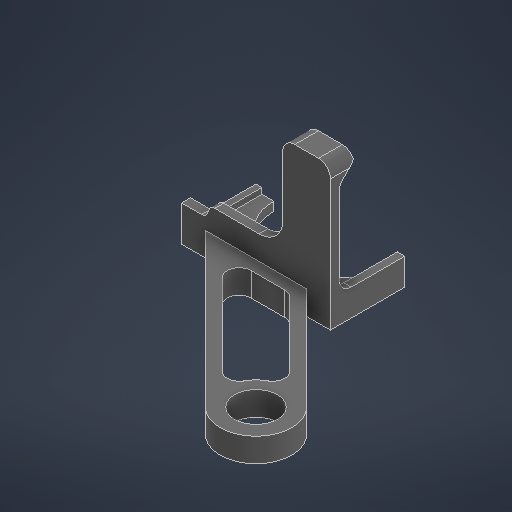
# Autodesk Inventor part: P_DroneCase
Saved by Autodesk Inventor 2026.2 (Build 302298000, 298)
## iProperties
Created: 2025-08-01
Part Number: P_DroneCase
Material: Generisch
Document SubType Name: Modeling
Designer: FAL
Density: 1 g/cm^3
Appearance: Vorgabe
Author: FAL
Autodesk Inventor part; units mm, degrees
ref_plane "YZ Plane" through (0, 0, 0) normal (1, 0, 0) x (0, 1, 0)
ref_plane "XZ Plane" through (0, 0, 0) normal (0, 1, 0) x (-1, 0, 0)
ref_plane "XY Plane" through (0, 0, 0) normal (0, 0, 1) x (1, 0, 0)
sketch "Skizze1" plane through (0, 0, 0) normal (0, 0, 1) x (1, 0, 0)
  line L0 (-25, 0) -> (25, 0)
  line L1 (25, 0) -> (25, -12.5)
  line L2 (25, -12.5) -> (-25, -12.5)
  line L3 (-25, -12.5) -> (-25, 0)
  line L4 (0, 0) -> (0, -12.5)
  dimension "d0" = 50
  dimension "d1" = 12.5
  constraints: 10 end point, 3 midpoint, 2 parallel, 1 horizontal, 1 perpendicular, 1 point on line
  measures "d0" distance of L1.end L2.end
  measures "d1" distance between parallel lines of L0 L2
extrude "Extrusion1" add sketch "Skizze1" along normal blind 24 contours L0 L1 L2 L4
sketch "Skizze24" plane through (0, 0, 0) normal (0, 0, 1) x (1, 0, 0)
  line L0 (0, 0) -> (33.9411, -33.9411) construction
  line L1 (4.2426, 4.2426) -> (38.1838, -29.6985)
  line L2 (29.6985, -38.1838) -> (-4.2426, -4.2426)
  arc A0 (4.2426, 4.2426) -> (-4.2426, -4.2426) centre (0, 0) ccw
  arc A1 (29.6985, -38.1838) -> (38.1838, -29.6985) centre (33.9411, -33.9411) ccw
  line L3 (0, 0) -> (0, -54.7704)
  line L4 (25, -12.5) -> (25, 0) projected
  line L5 (25, 0) -> (-45.4025, 0)
  point P0 (16.9706, -16.9706)
  point P1 (8.4853, 0)
  point P2 (-6, 0)
  point P3 (0, -8.4853)
  dimension "d137" = 45
  dimension "d138" = 48
  dimension "d139" = 12
  constraints: 12 end point, 4 point on circle, 4 tangent, 2 centre point, 1 horizontal, 1 midpoint, 1 parallel, 1 vertical
  measures "d137" angle of L3 L0
  measures "d138" distance of L0.start L0.end
  measures "d139" distance between parallel lines of L2 L1
extrude "Extrusion19" add sketch "Skizze24" along normal blind 4 contours L1 A1 L2 L3 L5
sketch "Skizze25" plane through (0, 0, 4) normal (0, 0, 1) x (1, 0, 0)
  arc A0 (29.6985, -38.1838) -> (38.1838, -29.6985) centre (33.9411, -33.9411) ccw projected
  circle A1 centre (33.9411, -33.9411) radius 3.575
  circle A2 centre (33.9411, -33.9411) radius 5.575
  line L0 (28.3667, -34.0236) -> (6.8431, -12.5)
  line L1 (0, -12.5) -> (25, -12.5) projected
  line L2 (18.1569, -12.5) -> (34.0236, -28.3667)
  line L3 (4.0147, -12.5) -> (29.6985, -38.1838) projected
  line L4 (38.1838, -29.6985) -> (20.9853, -12.5) projected
  line L5 (8.8431, -14.5) -> (20.1569, -14.5)
  point P0 (0, 0)
  point P1 (-35, -12.5)
  dimension "d142" = 7.15
  dimension "d143" = 2
  dimension "d144" = 2
  dimension "d145" = 2
  dimension "d149" = 2
  constraints: 6 end point, 4 parallel, 4 point on line, 2 centre point, 2 coincident, 2 point on circle
  measures "d142" diameter of A1
  measures "d143" distance between parallel lines of L3 L0
  measures "d144" distance between parallel lines of L4 L2
  measures "d145" radial gap between concentric circles of A1 A2
  measures "d149" distance between parallel lines of L1 L5
extrude "Extrusion20" cut sketch "Skizze25" against normal through all contours L5 L2 A2 L0 | A1
fillet "Rundung14" radius 2 4 edges at (28.3667, -34.0236, 2) (34.0236, -28.3667, 2) (8.8431, -14.5, 2) (20.1569, -14.5, 2)
sketch "Skizze26" plane through (25, -12.5, 0) normal (1, 0, 0) x (0, 0, -1)
  line L0 (0, 12.5) -> (-24, 12.5) projected
  line L1 (-24, 12.5) -> (-1.5, 12.5)
  line L2 (-1.5, 12.5) -> (-1.5, 1.5)
  line L3 (-1.5, 1.5) -> (-24, 1.5)
  line L4 (-24, 1.5) -> (-24, 12.5)
  line L5 (0, 0) -> (0, 12.5) projected
  line L6 (0, 0) -> (-24, 0) projected
  line L7 (-20.3, 1.5) -> (-22.8, 4)
  line L8 (-22.8, 4) -> (-24, 4)
  point P0 (-1.5, 12.5)
  dimension "d151" = 1.5
  dimension "d152" = 1.5
  dimension "d166" = 2.5
  dimension "d167" = 1.2
  dimension "d168" = 45
  constraints: 12 end point, 2 parallel, 2 perpendicular, 2 point on line, 1 horizontal
  measures "d151" distance between parallel lines of L5 L2
  measures "d152" distance between parallel lines of L6 L3
  measures "d166" distance between parallel lines of L3 L8
  measures "d167" distance of L7.end L8.end
  measures "d168" angle of L3 L7
extrude "Extrusion21" cut sketch "Skizze26" against normal blind 54.5 contours L2 L3 L7 L8 L4 L0
sketch "Skizze27" plane through (25, -11, 1.5) normal (0, 0, 1) x (1, 0, 0)
  line L0 (0, 11) -> (-25, 11) projected
  line L1 (-14, 11) -> (-11, 11) construction
  line L2 (-14, 19) -> (-11, 19)
  line L3 (-11, 3) -> (-14, 3)
  arc A0 (-14, 19) -> (-14, 3) centre (-14, 11) ccw
  arc A1 (-11, 3) -> (-11, 19) centre (-11, 11) ccw
  point P0 (-12.5, 11)
  point P1 (-3, 11)
  point P2 (-22, 11)
  dimension "d156" = 3
  dimension "d157" = 3
  dimension "d169" = 8
  constraints: 8 end point, 6 point on circle, 4 tangent, 2 centre point, 2 point on line, 1 midpoint, 1 parallel
  measures "d156" distance of L0.start point (-3, 11)
  measures "d157" distance of L0.end point (-22, 11)
  measures "d169" distance between parallel lines of L0 L3
extrude "Extrusion22" cut sketch "Skizze27" against normal blind 54.5
fillet "Rundung16" radius 2 1 edges at (12.5, -11, 1.5)
sketch "Skizze28" plane through (0, 0, 0) normal (0, 1, 0) x (-1, 0, 0)
  line L0 (0, 24) -> (-25, 24) projected
  line L1 (-17, 24) -> (5.438, 24)
  line L2 (5.438, 24) -> (5.438, 8)
  line L3 (5.438, 8) -> (-17, 8)
  line L4 (-17, 8) -> (-17, 24)
  line L5 (-25, 0) -> (-25, 24) projected
  line L6 (-4.0147, 4) -> (-29.6985, 4) projected
  line L7 (-4.9326, 8) -> (-4, 6)
  line L8 (-4, 6) -> (0, 6)
  line L9 (0, 20.3) -> (0, 3.5) projected
  point P0 (0, 0)
  point P1 (0, 8)
  dimension "d161" = 8
  dimension "d162" = 4
  dimension "d178" = 2
  dimension "d179" = 4
  dimension "d180" = 115
  constraints: 12 end point, 3 point on line, 2 horizontal, 2 parallel, 1 perpendicular
  measures "d161" distance between parallel lines of L5 L4
  measures "d162" distance between parallel lines of L6 L3
  measures "d178" distance between parallel lines of L6 L8
  measures "d179" distance from line of L9 L7.end
  measures "d180" angle of L8 L7
extrude "Extrusion23" cut sketch "Skizze28" against normal through all
fillet "Rundung17" radius 4 1 edges at (17, -11.75, 8)
fillet "Rundung18" radius 2 2 edges at (25, -10.5, 24) (17, -10.5, 24)
sketch "Skizze29" plane through (22, 0, 1.5) normal (0, 0, 1) x (1, 0, 0)
  line L0 (-22, -12.5) -> (-17.9853, -12.5) projected
  line L1 (-19, 0) -> (-22, 0) projected
  line L2 (-22, -12.5) -> (-21, -12.5)
  line L3 (-21, -12.5) -> (-21, 0)
  line L4 (-21, 0) -> (-22, 0)
  line L5 (-22, 0) -> (-22, -12.5)
  line L6 (3, 0) -> (0, 0) projected
  line L7 (3, -12.5) -> (1, -12.5) projected
  line L8 (3, 0) -> (2, 0)
  line L9 (2, 0) -> (2, -12.5)
  line L10 (2, -12.5) -> (3, -12.5)
  line L11 (3, -12.5) -> (3, 0)
  point P0 (-21, -12.5)
  point P1 (3, -12.5)
  point P2 (2, 0)
  dimension "d171" = 1
  dimension "d175" = 1
  constraints: 16 end point, 4 parallel, 2 horizontal, 2 perpendicular, 1 midpoint, 1 point on line
  measures "d171" distance between parallel lines of L5 L3
  measures "d175" distance between parallel lines of L11 L9
extrude "Extrusion24" add sketch "Skizze29" along normal blind 1 contours L5 L1 L3 L0
fillet "Rundung19" radius 2 1 edges at (21, -11, 20.3)
fillet "Rundung22" radius 1 2 edges at (4.9326, -11.75, 8) (4, -11.75, 6)
sketch "Skizze30" plane through (22, 0, 1.5) normal (0, 0, 1) x (1, 0, 0)
  line L0 (3, -12.5) -> (3, 0) projected
  line L1 (-1.0147, -12.5) -> (3, -12.5) projected
  line L2 (3, 0) -> (1.75, 0)
  line L3 (1.75, 0) -> (1.75, -12.5)
  line L4 (1.75, -12.5) -> (3, -12.5)
  line L5 (3, -12.5) -> (3, 0)
  point P0 (-22, 0)
  dimension "d182" = 1.25
  constraints: 8 end point, 2 parallel, 1 horizontal, 1 perpendicular, 1 point on line
  measures "d182" distance between parallel lines of L0 L3
extrude "Extrusion25" add sketch "Skizze30" along normal blind 3
fillet "Rundung23" radius 2 1 edges at (24.375, -11, 4.5)
